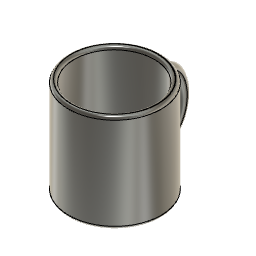
gyakorlati 5 pohar (Autodesk Fusion 360 design; units mm, degrees)
Autodesk Fusion 360 part; units mm, degrees
sketch "Sketch1" plane through (0, 0, 0) normal (0, 0, 1) x (1, 0, 0)
  circle A0 centre (0, 0) radius 75
  constraint coincident A0.centre origin
extrude "Extrude1" add sketch "Sketch1" along normal blind 160
sketch "Sketch2" plane through (0, 0, 0) normal (1, 0, 0) x (0, 1, 0)
  spline S0 degree 5 poles (65, 120) (66.1931, 121.5325) (68.5773, 124.3484) (72.148, 127.8246) (76.8975, 130.9584) (82.7951, 132.3601) (88.5915, 131.2697) (94.165, 127.7816) (99.3057, 122.109) (103.7425, 114.5719) (107.1889, 105.5686) (109.384, 95.5552) (110.1351, 85.0252) (109.3635, 74.4909) (107.15, 64.465) (103.6857, 55.4422) (99.2297, 47.8799) (94.0646, 42.1776) (88.4579, 38.6559) (82.6158, 37.5275) (76.6575, 38.8863) (71.8468, 41.9819) (68.223, 45.4273) (65.8001, 48.2215) (64.587, 49.743) knots 0 0 0 0 0 0 0.05 0.1 0.15 0.2 0.25 0.3 0.35 0.4 0.45 0.5 0.55 0.6 0.65 0.7 0.75 0.8 0.85 0.9 0.95 1 1 1 1 1 1
  point P0 (90, 130)
  point P1 (109.7554, 85.3182)
  point P2 (90, 40)
pipe "Pipe1" add diameter 15 path "Sketch2" along S0
hole "Hole1" at (-0.4365, -0.568, 160) direction (0, 0, -1) diameter 130 depth 150 tip angle 180 counterbore diameter 154 counterbore depth 1
fillet "Fillet1" radius 5 1 edges at (-69.9246, 27.1212, 159)
fillet "Fillet2" radius 5 1 edges at (-61.0378, 22.937, 159)
fillet "Fillet3" radius 5 1 edges at (-69.9246, -27.1212, 0)
